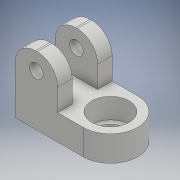
# Autodesk Inventor part: tiller rotation bracket
Saved by Autodesk Inventor 2017 (Build 210142000, 142)
## iProperties
Created: 2017-12-08
Part Number: tiller rotation bracket
Material: Generic
Document SubType Name: Modeling
Designer: RLanting
Density: 1 g/cm^3
Appearance: Default
Author: RLanting
Autodesk Inventor part; units mm, degrees
ref_plane "YZ Plane" through (0, 0, 0) normal (1, 0, 0) x (0, 1, 0)
ref_plane "XZ Plane" through (0, 0, 0) normal (0, 1, 0) x (-1, 0, 0)
ref_plane "XY Plane" through (0, 0, 0) normal (0, 0, 1) x (1, 0, 0)
sketch "Sketch1" plane through (0, 0, 0) normal (0, 0, 1) x (1, 0, 0)
  line L0 (0, 0) -> (-40, 0) construction
  line L1 (0, 16) -> (-40, 16)
  line L2 (-40, -16) -> (0, -16)
  arc A0 (0, -16) -> (0, 16) centre (0, 0) ccw
  arc A1 (-40, 16) -> (-40, -16) centre (-40, 0) ccw construction
  circle A2 centre (0, 0) radius 11
  line L3 (-40, 16) -> (-40, -16)
  point P0 (-20, 0)
  dimension "d0" = 22
  dimension "d1" = 5
  dimension "d2" = 40
  constraints: 10 end point, 4 point on circle, 4 tangent, 3 centre point, 1 coincident, 1 horizontal, 1 midpoint, 1 parallel, 1 vertical
  measures "d0" diameter of A2
  measures "d1" radial gap between concentric circles of A0 A2
  measures "d2" distance of L0.start L0.end
extrude "Extrusion1" add sketch "Sketch1" along normal blind 15
sketch "Sketch2" plane through (0, 0, 15) normal (0, 0, 1) x (1, 0, 0)
  line L0 (0, 16) -> (-40, 16) projected
  line L1 (-40, 16) -> (-15, 16)
  line L2 (-15, 16) -> (-15, 7.5)
  line L3 (-15, 7.5) -> (-40, 7.5)
  line L4 (-40, 7.5) -> (-40, 16)
  line L5 (-40, 16) -> (-40, -16) projected
  line L6 (-40, -16) -> (-15, -16)
  line L7 (-15, -16) -> (-15, -7.5)
  line L8 (-15, -7.5) -> (-40, -7.5)
  line L9 (-40, -7.5) -> (-40, -16)
  point P0 (0, 0)
  dimension "d5" = 25
  dimension "d6" = 15
  constraints: 16 end point, 4 parallel, 2 horizontal, 2 perpendicular, 1 collinear, 1 point on line
  measures "d5" distance of L2.end L3.end
  measures "d6" distance between parallel lines of L8 L3
extrude "Extrusion2" add sketch "Sketch2" along normal blind 25
sketch "Sketch3" plane through (-40, -16, 0) normal (0, -1, 0) x (1, 0, 0)
  line L0 (0, 15) -> (25, 15) projected
  line L1 (0, 40) -> (25, 40) construction
  line L2 (12.5, 40) -> (12.5, 30) construction
  circle A0 centre (12.5, 30) radius 4
  point P0 (40, 0)
  dimension "d9" = 8
  dimension "d10" = 10
  constraints: 2 end point, 1 centre point, 1 coincident, 1 midpoint, 1 vertical
  measures "d9" diameter of A0
  measures "d10" distance of L2.start L2.end
extrude "Extrusion3" cut sketch "Sketch3" against normal through all
fillet "Fillet1" radius 12 4 edges at (-15, 11.75, 40) (-40, 11.75, 40) (-15, -11.75, 40) (-40, -11.75, 40)
sketch "Sketch4" plane through (0, 0, 0) normal (0, 0, -1) x (-1, 0, 0)
  circle A0 centre (0, 0) radius 11 projected
  circle A1 centre (0, 0) radius 8
  dimension "d14" = 16
  constraints: 1 centre point, 1 coincident
  measures "d14" diameter of A1
extrude "Extrusion4" add sketch "Sketch4" against normal blind 3
body "Solid1"
